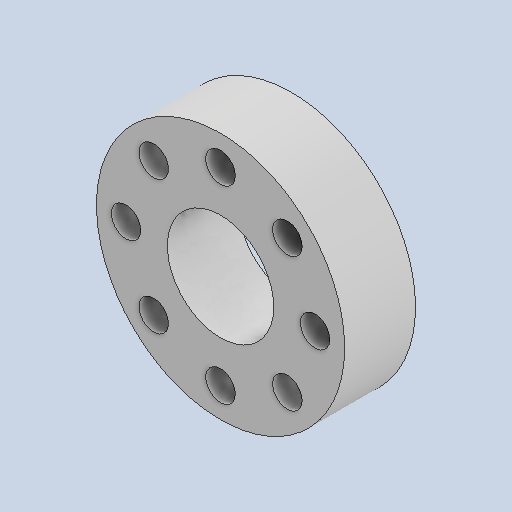
# Autodesk Inventor part: Motor_horn_mount
Saved by Autodesk Inventor 2022 (Build 260153000, 153)
## iProperties
Created: 2021-07-25
Part Number: Motor_horn_mount
Material: Generic
Document SubType Name: Modeling
Designer: exllu
Density: 1 g/cm^3
Appearance: Default
Author: exllu
Autodesk Inventor part; units mm, degrees
ref_plane "YZ Plane" through (0, 0, 0) normal (1, 0, 0) x (0, 1, 0)
ref_plane "XZ Plane" through (0, 0, 0) normal (0, 1, 0) x (-1, 0, 0)
ref_plane "XY Plane" through (0, 0, 0) normal (0, 0, 1) x (1, 0, 0)
sketch "Sketch1" plane through (0, 0, 0) normal (0, 0, 1) x (1, 0, 0)
  circle A0 centre (0, 0) radius 10.5
  line L0 (0, 0) -> (8, 0)
  circle A1 centre (8, 0) radius 1.25
  circle A2 centre (5.6569, 5.6569) radius 1.25
  circle A3 centre (0, 8) radius 1.25
  circle A4 centre (-5.6569, 5.6569) radius 1.25
  circle A5 centre (-8, 0) radius 1.25
  circle A6 centre (-5.6569, -5.6569) radius 1.25
  circle A7 centre (0, -8) radius 1.25
  circle A8 centre (5.6569, -5.6569) radius 1.25
  dimension "d0" = 21
  dimension "d1" = 8
  dimension "d2" = 2.5
  dimension "d5" = 360
  constraints: 11 coincident, 9 centre point, 2 end point, 1 horizontal, 31 other
  measures "d0" diameter of A0
  measures "d1" distance of L0.start L0.end
  measures "d2" diameter of A1
extrude "Extrusion1" add sketch "Sketch1" along normal blind 6
sketch "Sketch2" plane through (0, 0, 6) normal (0, 0, 1) x (1, 0, 0)
  circle A0 centre (0, 0) radius 4.5
  dimension "d9" = 9
  constraints: 1 centre point, 1 coincident
  measures "d9" diameter of A0
extrude "Extrusion2" cut sketch "Sketch2" against normal blind 6
body "Solid1"
